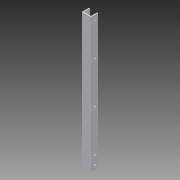
# Autodesk Inventor part: 18in C-Channel Front
Saved by Autodesk Inventor 2013 (Build 170138000, 138)
## iProperties
Created: 2013-01-08
Part Number: 18in C-Channel Front
Material: Aluminum 6061
Document SubType Name: Modeling
Designer: Naphat
Density: 1 g/cm^3
Author: Naphat
Autodesk Inventor part; units mm, degrees
ref_plane "YZ Plane" through (0, 0, 0) normal (1, 0, 0) x (0, 1, 0)
ref_plane "XZ Plane" through (0, 0, 0) normal (0, 1, 0) x (-1, 0, 0)
ref_plane "XY Plane" through (0, 0, 0) normal (0, 0, 1) x (1, 0, 0)
sketch "Sketch1" plane through (0, 0, 0) normal (0, 0, 1) x (1, 0, 0)
  line L0 (-16, 12.5) -> (-13, 12.5)
  line L1 (-13, 12.5) -> (-13, -9.5)
  line L2 (-13, -9.5) -> (13, -9.5)
  line L3 (13, -9.5) -> (13, 12.5)
  line L4 (13, 12.5) -> (16, 12.5)
  line L5 (16, 12.5) -> (16, -12.5)
  line L6 (16, -12.5) -> (-16, -12.5)
  line L7 (-16, -12.5) -> (-16, 12.5)
  point P0 (0, 0)
  dimension "d0" = 3
  dimension "d2" = 3
  dimension "d3" = 25
  dimension "d4" = 32
  dimension "d5" = 16
  dimension "d7" = 12.5
  dimension "d8" = 3
  dimension "d53" = 25
  constraints: 16 end point, 5 parallel, 1 collinear, 1 horizontal, 1 perpendicular
  measures "d0" distance of L0.start L0.end
  measures "d2" distance of L3.end L4.end
  measures "d3" distance of L6.end L0.start
  measures "d4" distance of L5.end L6.end
  measures "d5" distance from line of point (0, 0) L7
  measures "d7" distance from line of L6 point (0, 0)
  measures "d8" distance between parallel lines of L6 L2
  measures "d53" distance between parallel lines of L6 L4
extrude "Extrusion1" add sketch "Sketch1" against normal blind 482.6
sketch "Sketch12" plane through (16, -12.5, 0) normal (1, 0, 0) x (0, 0, -1)
  circle A0 centre (16, 14) radius 3.175 projected
  circle A1 centre (16, 14) radius 3.175
  circle A2 centre (466.6, 14) radius 3.175 projected
  circle A3 centre (466.6, 14) radius 3.175
  circle A4 centre (135, 14) radius 3.175 projected
  circle A5 centre (135, 14) radius 3.175
  circle A6 centre (434.6, 14) radius 3.175 projected
  circle A7 centre (284.8, 14) radius 3.175 projected
  point P0 (0, 12.5)
  constraints: 3 centre point, 3 coincident, 3 concentric
hole "Hole2" at (16, 1.5, -16) at (16, 1.5, -466.6) at (16, 1.5, -135) at (16, 1.5, -434.6) at (16, 1.5, -284.8) direction (-1, 0, 0) diameter 6.35 end through all
sketch "Sketch13" plane through (16, -12.5, 0) normal (1, 0, 0) x (0, 0, -1)
  circle A0 centre (351.875, 14.0056) radius 2 projected
  circle A1 centre (221.925, 14.0056) radius 2 projected
  point P0 (0, 12.5)
hole "Hole3" at (16, 1.5056, -351.875) at (16, 1.5056, -221.925) direction (-1, 0, 0) diameter 4 depth 3 tip angle 118
equation "\"d2\" = d0"
equation "\"d5\" = 0.5 * d4"
equation "\"d7\" = 0.5 * d3"
equation "\"d8\" = d0"
equation "\"d53\" = d3"
body "Solid1"
